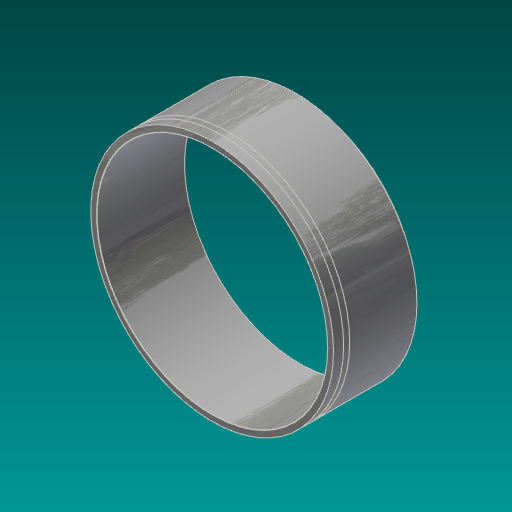
# Autodesk Inventor part: A1-19037-300-03 30in pipe
Saved by Autodesk Inventor 2017.3 (Build 213256000, 256)
## iProperties
Created: 2019-08-22
Part Number: A1-19037-300-03 30in pipe
Material: Steel, Mild
Document SubType Name: Modeling
Designer: GVD
Density: 7.85 g/cm^3
Appearance: Steel
Project: A1-19037--CNUL Albian CST laterals
Mass: 93965.7 g
Surface Area: 13521.7 cm^2
Volume: 11970.2 cm^3
Constructed By: Graeme_Van_Dongen
Project Name: CST laterals
Author: GVD
Autodesk Inventor part; units mm, degrees
ref_plane "YZ Plane" through (0, 0, 0) normal (1, 0, 0) x (0, 1, 0)
ref_plane "XZ Plane" through (0, 0, 0) normal (0, 1, 0) x (-1, 0, 0)
sketch "Sketch1" plane through (0, 0, 0) normal (0, 0, 1) x (1, 0, 0)
  circle A0 centre (0, 0) radius 381
  circle A1 centre (0, 0) radius 361.95
  dimension "d0" = 762
  dimension "d1" = 723.9
  constraints: 2 centre point, 2 coincident
  measures "d0" diameter of A0
  measures "d1" diameter of A1
extrude "Extrusion1" add sketch "Sketch1" along normal blind 275.4312
chamfer "Chamfer1" distance 17.4625 angle 37.5 1 edges at (-381, 0, 0) measured on face at (-374.402, -4.4582, 0)
ref_plane "Work Plane2" through (0, 0, 243.6812) normal (0, 0, 1) x (1, 0, 0)
ref_plane "Work Plane1" through (0, 0, 224.6312) normal (0, 0, 1) x (1, 0, 0)
split_face "Split1"
split_face "Split2"
chamfer "Chamfer2" distance 0.7937 angle 45 1 edges at (-361.95, 0, 275.4312)
body "Solid1"
